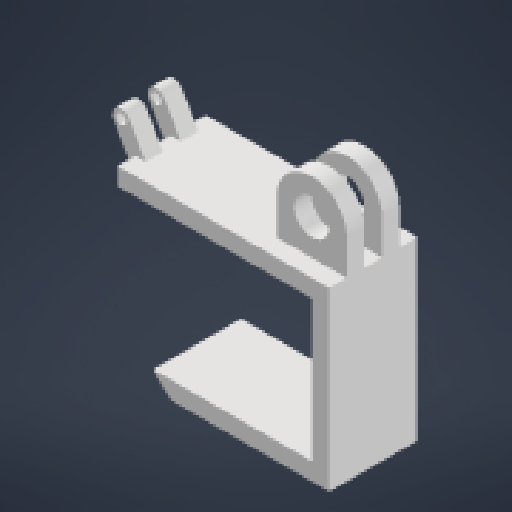
# Autodesk Inventor part: Claw New side
Saved by Autodesk Inventor 2023.6 (Build 276521000, 521)
## iProperties
Created: 2026-03-04
Part Number: Claw New side
Material: Generic
Document SubType Name: Modeling
Designer: user
Density: 1 g/cm^3
Appearance: Default
Author: user
Autodesk Inventor part; units mm, degrees
ref_plane "YZ Plane" through (0, 0, 0) normal (1, 0, 0) x (0, 1, 0)
ref_plane "XZ Plane" through (0, 0, 0) normal (0, 1, 0) x (-1, 0, 0)
ref_plane "XY Plane" through (0, 0, 0) normal (0, 0, 1) x (1, 0, 0)
sketch "Sketch1" plane through (0, 0, 0) normal (0, 0, 1) x (1, 0, 0)
  circle A0 centre (-31.2153, 30.6223) radius 1.5
  line L0 (22.8696, 23.547) -> (22.8696, 28.547)
  line L1 (-24.2436, 23.547) -> (22.8696, 23.547)
  line L2 (-24.2436, 23.547) -> (-29.0502, 31.8723)
  arc A1 (-29.0502, 31.8723) -> (-33.3804, 29.3723) centre (-31.2153, 30.6223) ccw
  line L3 (-33.3804, 29.3723) -> (-27.1304, 18.547)
  line L4 (27.8696, 18.547) -> (-27.1304, 18.547)
  line L5 (27.8696, -21.453) -> (27.8696, 18.547)
  line L6 (-17.1304, -21.453) -> (27.8696, -21.453)
  line L7 (-12.1304, -26.453) -> (-17.1304, -21.453)
  line L8 (32.8696, -26.453) -> (-12.1304, -26.453)
  line L9 (32.8696, 28.547) -> (32.8696, -26.453)
  arc A2 (32.8696, 28.547) -> (22.8696, 28.547) centre (27.8696, 28.547) ccw
  line L10 (27.8696, 18.547) -> (-27.1304, 18.547)
  line L11 (-24.2436, 23.547) -> (-27.1304, 23.547)
  line L12 (-27.1304, 18.547) -> (-27.1304, 23.547)
  line L13 (-27.1304, 23.547) -> (-24.2436, 23.547)
  line L14 (-24.2436, 23.547) -> (32.8696, 23.547)
  line L15 (32.8696, 28.547) -> (32.8696, -26.453)
  point P0 (0, 0)
  point P1 (-2.3882, 28.0958)
  point P2 (32.8696, 23.547)
  point P3 (22.8696, 23.547)
  dimension "d6" = 10
  dimension "d7" = 60
  dimension "d9" = 45
  dimension "d10" = 55
  dimension "d11" = 5
  dimension "d14" = 50
  dimension "d15" = 5
  dimension "d19" = 5
  dimension "d20" = 5
  constraints: 32 end point, 4 point on circle, 3 centre point, 2 point on line, 1 coincident, 1 perpendicular, 1 vertical
  measures "d6" distance between parallel lines of L9 L0
  measures "d7" distance between parallel lines of L9 L12
  measures "d9" distance of L6.start L5.start
  measures "d10" distance between parallel lines of L5 L12
  measures "d11" distance between parallel lines of L8 L6
  measures "d14" distance of L8.start L14.end
  measures "d15" radius of A2
  measures "d19" distance from line of L14 A2.centre
  measures "d20" distance between parallel lines of L4 L1
extrude "Extrusion1" add sketch "Sketch1" along normal mid plane 25 contours L14 L9 L8 L7 L6 L5 L4 L12 L11 L1
extrude "Extrusion2" add sketch "Sketch1" along normal mid plane 19 contours L11 L12 L3 A1 L2
extrude "Extrusion3" cut sketch "Sketch1" along normal mid plane 13 contours L0 A2 L9 L14 | L11 L12 L3 A1 L2
extrude "Extrusion5" add sketch "Sketch1" along normal mid plane 15 contours L0 A2 L9 L14
extrude "Extrusion6" cut sketch "Sketch1" along normal mid plane 5 contours L0 A2 L9 L14
sketch "Sketch3" plane through (0, 0, 7.5) normal (0, 0, 1) x (1, 0, 0)
  arc A0 (32.8696, 28.547) -> (22.8696, 28.547) centre (27.8696, 28.547) ccw projected
  circle A1 centre (27.8696, 28.547) radius 2.5
  point P0 (0, 0)
  dimension "d25" = 5
  constraints: 1 centre point, 1 coincident
  measures "d25" diameter of A1
extrude "Extrusion7" cut sketch "Sketch3" against normal through all
body "Solid1"
